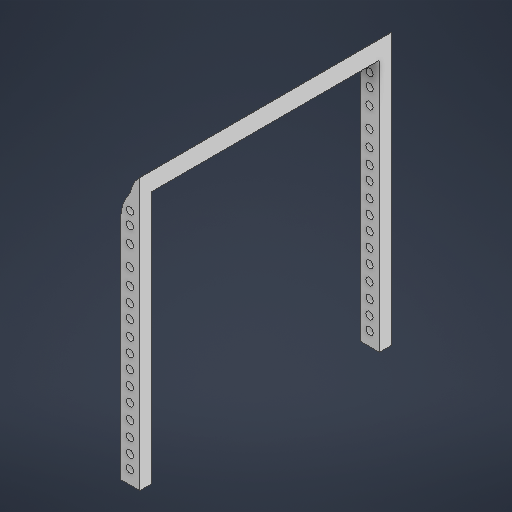
# Autodesk Inventor part: rails+scoop
Saved by Autodesk Inventor 2026.1 (Build 301233020, 233B)
## iProperties
Created: 2026-02-04
Part Number: rails+scoop
Material: Generic
Document SubType Name: Modeling
Designer: Dylan
Density: 1 g/cm^3
Appearance: Default
Author: Dylan
Autodesk Inventor part; units mm, degrees
ref_plane "YZ Plane" through (0, 0, 0) normal (1, 0, 0) x (0, 1, 0)
ref_plane "XZ Plane" through (0, 0, 0) normal (0, 1, 0) x (-1, 0, 0)
ref_plane "XY Plane" through (0, 0, 0) normal (0, 0, 1) x (1, 0, 0)
sketch "Sketch1" plane through (0, 0, 0) normal (0, 1, 0) x (-1, 0, 0)
  line L0 (0, 0) -> (-5.3, 0)
  line L1 (-5.3, 0) -> (-5.3, -3.3)
  line L2 (-5.3, -3.3) -> (0, -3.3)
  line L3 (0, -3.3) -> (0, 0)
  line L4 (0, -66.3) -> (-5.3, -66.3)
  line L5 (-5.3, -66.3) -> (-5.3, -69.6)
  line L6 (-5.3, -69.6) -> (0, -69.6)
  line L7 (0, -69.6) -> (0, -66.3)
  dimension "d0" = 5.3
  dimension "d1" = 3.3
  dimension "d2" = 63
  dimension "d3" = 5.3
  dimension "d4" = 3.3
  constraints: 16 end point, 4 parallel, 2 horizontal, 2 perpendicular
  measures "d0" distance of L2.end L1.end
  measures "d1" distance of L1.end L0.end
  measures "d2" distance of L2.end L4.start
  measures "d3" distance of L6.end L5.end
  measures "d4" distance of L5.end L4.end
sketch "Sketch1 outline for Rails" plane through (0, 0, 0) normal (0, 1, 0) x (-1, 0, 0)
  line L0 (0, -66.3) -> (-5.3, -66.3)
  line L1 (0, -69.6) -> (0, -66.3)
  line L2 (-5.3, -69.6) -> (0, -69.6)
  line L3 (-5.3, -66.3) -> (-5.3, -69.6)
  line L4 (0, 0) -> (-5.3, 0)
  line L5 (0, -3.3) -> (0, 0)
  line L6 (-5.3, -3.3) -> (0, -3.3)
  line L7 (-5.3, 0) -> (-5.3, -3.3)
extrude "Rails" add sketch "Sketch1 outline for Rails" along normal blind 70
sketch "Sketch2" plane through (0, 70, 0) normal (0, 1, 0) x (1, 0, 0)
  line L0 (0, 0) -> (5.3, 0) projected
  line L1 (5.3, 66.3) -> (5.3, 69.6) projected
  line L2 (2.65, 0) -> (5.3, 0)
  line L3 (5.3, 0) -> (5.3, 69.6)
  line L4 (5.3, 69.6) -> (2.65, 69.6)
  line L5 (2.65, 69.6) -> (2.65, 0)
  constraints: 8 end point, 2 parallel, 1 horizontal, 1 midpoint, 1 perpendicular
sketch "Sketch2 outline for Extrusion2" plane through (0, 70, 0) normal (0, 1, 0) x (1, 0, 0)
  line L0 (5.3, 69.6) -> (2.65, 69.6)
  line L1 (5.3, 66.3) -> (5.3, 69.6)
  line L2 (5.3, 0) -> (5.3, 66.3)
  line L3 (2.65, 0) -> (5.3, 0)
  line L4 (2.65, 69.6) -> (2.65, 0)
extrude "Extrusion2" add sketch "Sketch2 outline for Extrusion2" along normal blind 5
chamfer "Chamfer1" distance 2.6 angle 45 1 edges at (2.65, 75, -34.8)
fillet "Scoop lip" radius 9 1 edges at (2.65, 72.4, -34.8)
fillet "Purely Aesthetics" radius 12 2 edges at (0, 70, -1.65) (0, 70, -67.95)
sketch "Sketch4" plane through (0, 0, 0) normal (0, 0, 1) x (1, 0, 0)
  circle A0 centre (2.577408, 3.76) radius 1
  circle A1 centre (2.577408, 7.447823) radius 1
  circle A2 centre (2.577408, 11.422475) radius 1
  circle A3 centre (2.577408, 15.602007) radius 1
  circle A4 centre (2.577408, 19.740564) radius 1
  circle A5 centre (2.577408, 23.674241) radius 1
  circle A6 centre (2.577408, 27.68987) radius 1
  circle A7 centre (2.577408, 31.541595) radius 1
  circle A8 centre (2.577408, 35.516248) radius 1
  circle A9 centre (2.577408, 39.736756) radius 1
  circle A10 centre (2.577408, 43.547506) radius 1
  circle A11 centre (2.577408, 47.727037) radius 1
  circle A12 centre (2.577408, 52.234376) radius 1
  circle A13 centre (2.577408, 57.766109) radius 1
  circle A14 centre (2.577408, 62.191496) radius 1
  circle A15 centre (2.577408, 65.715415) radius 1
  point P0 (0, 0)
  dimension "d14" = 2
  dimension "d15" = 2
  dimension "d16" = 2
  dimension "d17" = 2
  dimension "d18" = 2
  dimension "d19" = 2
  dimension "d20" = 2
  dimension "d21" = 2
  dimension "d22" = 2
  dimension "d23" = 2
  dimension "d24" = 2
  dimension "d25" = 2
  dimension "d26" = 2
  dimension "d27" = 2
  dimension "d28" = 2
  dimension "d29" = 2
  constraints: 16 centre point
  measures "d14" diameter of A0
  measures "d15" diameter of A1
  measures "d16" diameter of A2
  measures "d17" diameter of A3
  measures "d18" diameter of A4
  measures "d19" diameter of A5
  measures "d20" diameter of A6
  measures "d21" diameter of A7
  measures "d22" diameter of A8
  measures "d23" diameter of A9
  measures "d24" diameter of A10
  measures "d25" diameter of A11
  measures "d26" diameter of A12
  measures "d27" diameter of A13
  measures "d28" diameter of A14
  measures "d29" diameter of A15
sketch "Sketch4 outline for Mesh Mounting Holes" plane through (0, 0, 0) normal (0, 0, 1) x (1, 0, 0)
  circle A0 centre (2.577408, 65.715415) radius 1
  circle A1 centre (2.577408, 62.191496) radius 1
  circle A2 centre (2.577408, 57.766109) radius 1
  circle A3 centre (2.577408, 52.234376) radius 1
  circle A4 centre (2.577408, 47.727037) radius 1
  circle A5 centre (2.577408, 43.547506) radius 1
  circle A6 centre (2.577408, 39.736756) radius 1
  circle A7 centre (2.577408, 35.516248) radius 1
  circle A8 centre (2.577408, 31.541595) radius 1
  circle A9 centre (2.577408, 27.68987) radius 1
  circle A10 centre (2.577408, 23.674241) radius 1
  circle A11 centre (2.577408, 19.740564) radius 1
  circle A12 centre (2.577408, 15.602007) radius 1
  circle A13 centre (2.577408, 11.422475) radius 1
  circle A14 centre (2.577408, 7.447823) radius 1
  circle A15 centre (2.577408, 3.76) radius 1
extrude "Mesh Mounting Holes" cut sketch "Sketch4 outline for Mesh Mounting Holes" against normal blind 70
body "Solid1"
